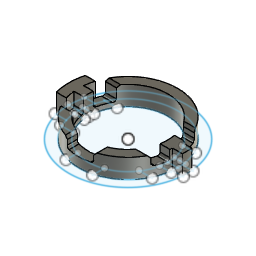
Toyota_Steering_Wheel_SRS_Adapter (Autodesk Fusion 360 design; units mm, degrees)
Autodesk Fusion 360 part; units mm, degrees
note: some values were not read from the file. Chosen so that the rebuilt part matches the saved one: which pieces of a blend or face edit are solid. Set by a fixed rule: which sketch regions a step uses.
sketch "sketch_v1" plane through (0, 0, 0) normal (0, 0, 1) x (1, 0, 0)
  line L0 (16.25, 0) -> (21, 0)
  line L1 (-21, -0.0002) -> (-16.25, -0.0002)
  line L2 (-20.9035, 2.0104) -> (-16.1252, 2.0104)
  line L3 (16.0565, 3) -> (20.8507, 3)
  line L4 (-18.9731, 9.0011) -> (-13.5293, 9.0011)
  line L5 (18.9737, 9) -> (13.5301, 9)
  line L6 (-18.9731, -9.0015) -> (-13.5293, -9.0015)
  line L7 (-20.9035, -2.0107) -> (-16.1252, -2.0107)
  line L8 (18.9737, -9) -> (13.5301, -9)
  line L9 (16.0565, -3) -> (20.8507, -3)
  line L10 (-21, -0.0002) -> (-25, -0.0002)
  line L11 (24.9199, 2) -> (20.4022, 2)
  line L12 (24.9199, -2) -> (20.4022, -2)
  line L13 (-24.2693, 5.9997) -> (-19.6024, 5.9997)
  line L14 (-24.2693, -6) -> (-19.6024, -6)
  line L15 (5.5289, -20.2591) -> (5.5289, -15.2805)
  line L16 (-5.4703, -20.275) -> (-5.4703, -15.3016)
  line L17 (-19.6024, -6) -> (-19.6023, -6)
  line L18 (-18.8624, 9.0011) -> (-18.9731, 9.0011)
  line L19 (-19.9, -2) -> (-19.9, -2.1)
  line L20 (-19.4745, 2.0104) -> (-19.4745, 2.1104)
  line L21 (18.4536, 3) -> (18.4536, 3.1)
  circle A0 centre (0, 0) radius 20.5
  circle A1 centre (0, 0) radius 16.5
  circle A2 centre (0, 0) radius 24.5
  dimension "d61" = 0.1
  dimension "d62" = 0.1
  dimension "d63" = 0.1
  dimension "d84" = 41
  dimension "d92" = 33
  dimension "d93" = 49
  constraint horizontal L0
  constraint parallel L0 L1
  constraint symmetric L1 L2.start L7.start
  constraint symmetric L1 L2.end L7.end
  constraint symmetric L1 L4.start L6.start
  constraint symmetric L1 L4.end L6.end
  constraint symmetric L0 L3.start L9.start
  constraint symmetric L0 L3.end L9.end
  constraint symmetric L0 L5.start L8.start
  constraint symmetric L0 L5.end L8.end
  constraint horizontal L10
  constraint symmetric L10 L13.start L14.start
  constraint symmetric L10 L13.end L14.end
  constraint vertical L16
  constraint horizontal L11
  constraint horizontal L12
  constraint horizontal L13
  constraint horizontal L6
  constraint horizontal L7
  constraint horizontal L8
  constraint horizontal L9
  constraint vertical L15
  constraint parallel L14 L17
  constraint coincident L4 L18.start
  constraint perpendicular L7 L19
  constraint coincident L2 L20.start
  constraint perpendicular L2 L20
  constraint midpoint L3 L21.start
  constraint perpendicular L3 L21
  constraint coincident L11.end A0
  constraint coincident L12.end A0
  constraint coincident L17.end A0
  constraint coincident L13.end A0
  constraint concentric A0 A2
  measures "d61" distance of L19.start L19.end
  measures "d62" distance of L20.start L20.end
  measures "d63" distance of L21.start L21.end
  measures "d84" diameter of A0
  measures "d92" diameter of A1
  measures "d93" diameter of A2
combine "Combine2" [no effect]
combine "Combine3" [no effect]
extrude "Extrude27" add sketch "sketch_v1" along normal blind 8 contours L0 L3 A0 A1 | L0 L9 A0 A1 | L11 L12 A0 A2 | L4 L5 A0 A1 | L8 L15 A0 A1 | L1 L10 L13 A0 A2 | L1 L10 L14 A0 A2 | L1 L2 A0 A1 | L6 L16 A0 A1 | L1 L7 A0 A1 makes body 1 at (-17.9747, -9.8569, 2.6667) makes body 2 at (-15.6445, 13.2477, 5.3333) makes body 3 at (-23.9812, 5.0154, 2.6667) makes body 4 at (13.846, -15.1175, 2.6667) makes body 5 at (16.415, -1.6731, 5.3333)
extrude "Extrude28" add sketch "sketch_v1" along normal blind 2 contours L2 L4 A0 A1 | L6 L7 A0 A1 bodies 1 2 3
extrude "Extrude29" add sketch "sketch_v1" along normal blind 4 contours L3 L5 A0 A1 | L8 L9 A0 A1 | L15 L16 A0 A1 bodies 1 4 5
chamfer "Chamfer1" distance 1 angle 45 6 edges at (5.5289, -17.6432, 8) (-5.4703, -17.6618, 8) (-16.1232, -9.0015, 8) (-16.1234, 9.0011, 8) (16.124, -9, 8) (16.124, 9, 8) on bodies 1
move_face "OffsetFaces2" offset -1 1 faces at (12.4383, 10.8415, 4) on bodies 1
fillet "Fillet1" radius 1 10 edges at (-18.8927, 2.0104, 2) (-18.8926, -2.0107, 2) (18.7601, 3, 4) (18.7601, -3, 4) (16.7135, -9, 4) (16.7135, 9, 4) (-16.7129, 9.0011, 2) (-16.7127, -9.0015, 2) (-5.4703, -18.1899, 4) (5.5289, -18.172, 4) on bodies 1
move_face "OffsetFaces3" offset 1 1 faces at (-7.695, -15.7174, 4.2988) on bodies 1
